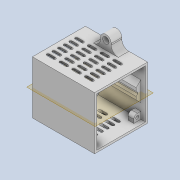
# Autodesk Inventor part: obudowa_WIZ2
Saved by Autodesk Inventor 2021 (Build 250183000, 183)
## iProperties
Created: 2025-11-29
Part Number: obudowa_WIZ2
Material: Generic
Document SubType Name: Modeling
Designer: huber
Density: 1 g/cm^3
Appearance: Default
Author: huber
Autodesk Inventor part; units mm, degrees
ref_plane "YZ Plane" through (0, 0, 0) normal (1, 0, 0) x (0, 1, 0)
ref_plane "XY Plane" through (0, 0, 0) normal (0, 0, 1) x (1, 0, 0)
sketch "Sketch1" plane through (0, 0, 0) normal (1, 0, 0) x (0, 1, 0)
  line L0 (37.5, 37.5) -> (-37.5, 37.5)
  line L1 (-37.5, 37.5) -> (-37.5, -37.5)
  line L2 (-37.5, -37.5) -> (37.5, -37.5)
  line L3 (37.5, -37.5) -> (37.5, 37.5)
  line L4 (37.5, 37.5) -> (-37.5, -37.5) construction
  line L5 (-37.5, 37.5) -> (37.5, -37.5) construction
  line L6 (34.5, 34.5) -> (-34.5, 34.5)
  line L7 (-34.5, 34.5) -> (-34.5, -34.5)
  line L8 (-34.5, -34.5) -> (34.5, -34.5)
  line L9 (34.5, -34.5) -> (34.5, 34.5)
  line L10 (34.5, 34.5) -> (-32.538, -32.538) construction
  line L11 (-34.5, 34.5) -> (32.4964, -32.4964) construction
  line L12 (-52.5, 0) -> (52.5, 0) projected
  line L13 (0, -52.5) -> (0, 52.5) projected
  line L14 (-14, 34.5) -> (-7.5, 28)
  line L15 (-7.5, 28) -> (7.5, 28)
  line L16 (7.5, 28) -> (14, 34.5)
  line L17 (-14, -34.5) -> (-7.5, -28)
  line L18 (-7.5, -28) -> (7.5, -28)
  line L19 (7.5, -28) -> (14, -34.5)
  line L20 (-3.15, 28) -> (-0.9, 30.25)
  line L21 (-0.9, 30.25) -> (0.9, 30.25)
  line L22 (0.9, 30.25) -> (3.15, 28)
  line L23 (-3.15, -28) -> (-0.9, -30.25)
  line L24 (-0.9, -30.25) -> (0.9, -30.25)
  line L25 (0.9, -30.25) -> (3.15, -28)
  point P0 (0, 0)
  dimension "d0" = 75
  dimension "d1" = 75
  dimension "d2" = 3
  dimension "d4" = 45
  dimension "d5" = 60.5
  dimension "d6" = 1.8
  dimension "d7" = 1.8
  dimension "d8" = 56
  dimension "d9" = 15
  dimension "d10" = 15
  dimension "d48" = 3
  dimension "d49" = 3
  dimension "d50" = 3
  constraints: 48 end point, 10 point on line, 6 parallel, 6 perpendicular, 4 horizontal, 2 midpoint, 6 other
  measures "d0" distance of L1.end L2.end
  measures "d1" distance of L0.end L1.end
  measures "d2" distance between parallel lines of L2 L8
  measures "d4" angle of L15 L22
  measures "d5" distance between parallel lines of L21 L24
  measures "d6" distance of L24.end L23.end
  measures "d7" distance of L21.end L20.end
  measures "d8" distance between parallel lines of L18 L15
  measures "d9" distance of L14.end L15.end
  measures "d10" distance of L18.end L17.end
  measures "d48" distance between parallel lines of L9 L3
  measures "d49" distance between parallel lines of L0 L6
  measures "d50" distance between parallel lines of L1 L7
extrude "Extrusion1" add sketch "Sketch1" along normal blind 85 contours L3 L12 L9 L6 L13 L0 | L13 L6 L7 L12 L1 L0 | L3 L2 L13 L8 L9 L12 | L13 L21 L20 L15 L14 L6 | L6 L16 L15 L22 L21 L13 | L12 L7 L8 L13 L2 L1 | L13 L24 L25 L18 L19 L8 | L8 L17 L18 L23 L24 L13
extrude "Extrusion2" add sketch "Sketch1" against normal blind 3
sketch "Sketch3" plane through (85, -37.5, -37.5) normal (0, -1, 0) x (1, 0, 0)
  line L0 (-88, 75) -> (0, 75) projected
  line L1 (-42.5, 75) -> (-42.5, 0) construction
  line L2 (0, 0) -> (-88, 0) projected
  line L3 (0, 75) -> (0, 0) projected
  point P0 (-85, 37.5)
  dimension "d16" = 42.5
  constraints: 2 end point, 2 point on line, 1 vertical
  measures "d16" distance between parallel lines of L3 L1
ref_plane "Work Plane1" through (42.5, -37.5, 37.5) normal (0.7071068, -0.7071068, 0) x (0, 0, -1)
sketch "Sketch5" plane through (42.5, -37.5, 37.5) normal (0.7071068, -0.7071068, 0) x (0, 0, -1)
  line L0 (0, 0) -> (75, 0) construction
  line L1 (37.5, 0) -> (37.5, 3.2791) construction
  line L2 (37.5, 0) -> (37.5, 13.5441)
  line L3 (37.5, 0) -> (37.5, 5) construction
  line L4 (39.5, 0) -> (39.5, 5)
  line L5 (35.5, 5) -> (35.5, 0)
  arc A0 (35.5, 0) -> (39.5, 0) centre (37.5, 0) ccw
  arc A1 (39.5, 5) -> (35.5, 5) centre (37.5, 5) ccw
  point P0 (37.5, -3.5355)
  point P1 (37.5, 2.5)
  dimension "d19" = 4
  dimension "d20" = 5
  constraints: 12 end point, 4 point on circle, 4 tangent, 2 centre point, 2 midpoint, 2 vertical, 1 parallel, 1 point on line
  measures "d19" distance between parallel lines of L4 L5
  measures "d20" distance of L1.start L3.end
extrude "Extrusion3" cut sketch "Sketch5" against normal mid plane 33
pattern_linear "Rectangular Pattern1" count 6 spacing 8 along (0, 0, 1) count 4 spacing 18 along (-1, 0, 0) of "Extrusion3" first direction both ways yes second direction both ways yes
mirror "Mirror1" about plane through (0, 0, 0) normal (0, 1, 0) of "Extrusion3", "Rectangular Pattern1"
sketch "Sketch6" plane through (-3, 0, 0) normal (-1, 0, 0) x (0, 0, 1)
  line L0 (0, 52.5) -> (0, -52.5) projected
  line L1 (-34.5, -14) -> (-34.5, -34.5) projected
  line L2 (-28, -7.5) -> (-34.5, -14) projected
  line L3 (-28, -3.15) -> (-28, -7.5) projected
  line L4 (-30.25, -0.9) -> (-28, -3.15) projected
  line L5 (-30.25, 0.9) -> (-30.25, -0.9) projected
  line L6 (-28, 3.15) -> (-30.25, 0.9) projected
  line L7 (-28, 7.5) -> (-28, 3.15) projected
  line L8 (-34.5, 14) -> (-28, 7.5) projected
  line L9 (-34.5, 34.5) -> (-34.5, 14) projected
  line L10 (34.5, 34.5) -> (-34.5, 34.5) projected
  line L11 (34.5, 14) -> (34.5, 34.5) projected
  line L12 (28, 7.5) -> (34.5, 14) projected
  line L13 (28, 3.15) -> (28, 7.5) projected
  line L14 (30.25, 0.9) -> (28, 3.15) projected
  line L15 (30.25, -0.9) -> (30.25, 0.9) projected
  line L16 (28, -3.15) -> (30.25, -0.9) projected
  line L17 (28, -7.5) -> (28, -3.15) projected
  line L18 (34.5, -14) -> (28, -7.5) projected
  line L19 (34.5, -34.5) -> (34.5, -14) projected
  line L20 (-34.5, -34.5) -> (34.5, -34.5) projected
  point P0 (0, 0)
extrude "Extrusion4" cut sketch "Sketch6" against normal blind 33
ref_plane "Work Plane2" through (78.5, 0, 0) normal (1, 0, 0) x (0, 0, -1)
sketch "Sketch7" plane through (78.5, 0, 0) normal (1, 0, 0) x (0, 0, -1)
  line L0 (37.5, -37.5) -> (37.5, 37.5) projected
  line L1 (37.5, 37.5) -> (-37.5, 37.5) projected
  line L2 (-37.5, 37.5) -> (-37.5, -37.5) projected
  line L3 (-37.5, -37.5) -> (37.5, -37.5) projected
  line L4 (34.5, -34.5) -> (-34.5, -34.5) projected
  line L5 (-34.5, -34.5) -> (-34.5, -14) projected
  line L6 (-34.5, -14) -> (-28, -7.5) projected
  line L7 (-28, -7.5) -> (-28, -3.15) projected
  line L8 (-28, -3.15) -> (-30.25, -0.9) projected
  line L9 (-30.25, -0.9) -> (-30.25, 0.9) projected
  line L10 (-30.25, 0.9) -> (-28, 3.15) projected
  line L11 (-28, 3.15) -> (-28, 7.5) projected
  line L12 (-28, 7.5) -> (-34.5, 14) projected
  line L13 (-34.5, 14) -> (-34.5, 34.5) projected
  line L14 (-34.5, 34.5) -> (34.5, 34.5) projected
  line L15 (34.5, 34.5) -> (34.5, 14) projected
  line L16 (34.5, 14) -> (28, 7.5) projected
  line L17 (28, 7.5) -> (28, 3.15) projected
  line L18 (28, 3.15) -> (30.25, 0.9) projected
  line L19 (30.25, 0.9) -> (30.25, -0.9) projected
  line L20 (30.25, -0.9) -> (28, -3.15) projected
  line L21 (28, -3.15) -> (28, -7.5) projected
  line L22 (28, -7.5) -> (34.5, -14) projected
  line L23 (34.5, -14) -> (34.5, -34.5) projected
  circle A0 centre (-29.5, 29.5) radius 2.15
  line L24 (-25.3431, 29.5) -> (-27.4215, 25.9)
  line L25 (-27.4215, 25.9) -> (-31.5785, 25.9)
  line L26 (-31.5785, 25.9) -> (-33.6569, 29.5)
  line L27 (-33.6569, 29.5) -> (-31.5785, 33.1)
  line L28 (-31.5785, 33.1) -> (-27.4215, 33.1)
  line L29 (-27.4215, 33.1) -> (-25.3431, 29.5)
  line L30 (-34.5, 34.5) -> (34.5, 34.5) projected
  circle A1 centre (-29.5, 29.5) radius 5
  line L31 (-24.5, 29.5) -> (-24.5, 34.5)
  line L32 (-29.5, 24.5) -> (-34.5, 24.5)
  line L33 (-34.5, 14) -> (-34.5, 34.5) projected
  circle A2 centre (29.5, -29.5) radius 5
  line L34 (25.3431, -29.5) -> (27.4215, -25.9)
  line L35 (27.4215, -25.9) -> (31.5785, -25.9)
  line L36 (31.5785, -25.9) -> (33.6569, -29.5)
  line L37 (33.6569, -29.5) -> (31.5785, -33.1)
  line L38 (31.5785, -33.1) -> (27.4215, -33.1)
  line L39 (27.4215, -33.1) -> (25.3431, -29.5)
  circle A3 centre (29.5, -29.5) radius 2.15
  line L40 (29.5, -24.5) -> (34.5, -24.5)
  line L41 (24.5, -29.5) -> (24.5, -34.5)
  line L42 (34.5, -14) -> (34.5, -34.5) projected
  point P0 (0, 0)
  point P1 (-34.5, 24.5)
  point P2 (-34.5, 29.5)
  point P3 (-29.5, 34.5)
  dimension "d33" = 4.3
  dimension "d34" = 5
  dimension "d35" = 5
  dimension "d36" = 7.2
  dimension "d41" = 5
  dimension "d42" = 5
  dimension "d43" = 7.2
  dimension "d44" = 4.3
  constraints: 32 end point, 6 tangent, 4 centre point, 4 coincident, 4 point on circle, 4 point on line, 2 parallel, 2 perpendicular, 1 horizontal, 1 vertical, 26 other
  measures "d33" diameter of A0
  measures "d34" distance from line of L14 A0.centre
  measures "d35" distance from line of L13 A0.centre
  measures "d36" distance between parallel lines of L25 L28
  measures "d41" distance from line of L23 A2.centre
  measures "d42" distance from line of A2.centre L4
  measures "d43" distance between parallel lines of L38 L35
  measures "d44" diameter of A3
extrude "Extrusion5" add sketch "Sketch7" against normal blind 8 contours L41 A2 L4 | A2 L23 L4 | A2 | A2 L40 L23 | L13 A1 L32 | L13 L14 A1 | A1 | L14 L31 A1
extrude "Extrusion6" add sketch "Sketch7" against normal blind 4 contours L24 L25 L26 L27 L28 L29 | L34 L35 L36 L37 L38 L39
ref_plane "Work Plane3" through (0, 37.5, -37.5) normal (0, -0.7071068, -0.7071068) x (1, 0, 0)
sketch "Sketch8" plane through (85, 0, 0) normal (1, 0, 0) x (0, 0, -1)
  line L0 (37.5, -37.5) -> (37.5, 37.5) projected
  line L1 (37.5, -37.5) -> (37.5, 37.5) projected
  line L2 (37.5, 37.5) -> (-37.5, 37.5) projected
  line L3 (-37.5, 37.5) -> (-37.5, -37.5) projected
  line L4 (-37.5, -37.5) -> (37.5, -37.5) projected
  line L5 (34.5, -34.5) -> (-34.5, -34.5) projected
  line L6 (-34.5, -34.5) -> (-34.5, -14) projected
  line L7 (-34.5, -14) -> (-28, -7.5) projected
  line L8 (-28, -7.5) -> (-28, -3.15) projected
  line L9 (-28, -3.15) -> (-30.25, -0.9) projected
  line L10 (-30.25, -0.9) -> (-30.25, 0.9) projected
  line L11 (-30.25, 0.9) -> (-28, 3.15) projected
  line L12 (-28, 3.15) -> (-28, 7.5) projected
  line L13 (-28, 7.5) -> (-34.5, 14) projected
  line L14 (-34.5, 14) -> (-34.5, 34.5) projected
  line L15 (-34.5, 34.5) -> (34.5, 34.5) projected
  line L16 (34.5, 34.5) -> (34.5, 14) projected
  line L17 (34.5, 14) -> (28, 7.5) projected
  line L18 (28, 7.5) -> (28, 3.15) projected
  line L19 (28, 3.15) -> (30.25, 0.9) projected
  line L20 (30.25, 0.9) -> (30.25, -0.9) projected
  line L21 (30.25, -0.9) -> (28, -3.15) projected
  line L22 (28, -3.15) -> (28, -7.5) projected
  line L23 (28, -7.5) -> (34.5, -14) projected
  line L24 (34.5, -14) -> (34.5, -34.5) projected
  line L25 (28, -7.5) -> (34.5, -14) projected
  line L26 (34.5, -14) -> (34.5, 14)
  line L27 (-34.5, -14) -> (-34.5, 14)
  point P0 (0, 0)
  constraints: 4 end point, 1 vertical
extrude "Extrusion8" cut sketch "Sketch8" against normal up to surface (6.5 mm away) contours L23 L22 L21 L20 L19 L18 L17 L26 | L27 L13 L12 L11 L10 L9 L8 L7
sketch "Sketch12" plane through (85, -37.5, -37.5) normal (0, 0, -1) x (-1, 0, 0)
  line L0 (88, 75) -> (0, 75) projected
  line L1 (0, 0) -> (0, 75) projected
  line L2 (0, 0) -> (88, 0) projected
  line L3 (88, 75) -> (88, 0) projected
  line L4 (88, 75) -> (0, 75) projected
  line L5 (44, 75) -> (44, 0)
  circle A0 centre (44, 87) radius 7.5
  line L6 (51.5, 87) -> (51.5, 75)
  line L7 (88, 75) -> (0, 75) projected
  line L8 (36.5, 87) -> (36.5, 75)
  point P0 (85, 37.5)
  dimension "d80" = 15
  dimension "d81" = 12
  constraints: 6 end point, 3 point on line, 2 midpoint, 2 perpendicular, 2 point on circle, 2 tangent, 1 centre point, 1 parallel
  measures "d80" diameter of A0
  measures "d81" distance from line of A0.centre L0
extrude "Extrusion10" add sketch "Sketch12" against normal blind 15 contours L0 L8 A0 L6 | A0
fillet "Fillet3" radius 10 2 edges at (33.5, 37.5, -30) (48.5, 37.5, -30)
sketch "Sketch13" plane through (85, -37.5, -22.5) normal (0, 0, 1) x (1, 0, 0)
  line L0 (-36.5, 85) -> (-36.5, 87) projected
  arc A0 (-36.5, 87) -> (-51.5, 87) centre (-44, 87) ccw projected
  line L1 (-51.5, 87) -> (-51.5, 85) projected
  arc A1 (-61.5, 75) -> (-51.5, 85) centre (-61.5, 85) ccw projected
  line L2 (-26.5, 75) -> (-61.5, 75) projected
  arc A2 (-36.5, 85) -> (-26.5, 75) centre (-26.5, 85) ccw projected
  point P0 (-85, 37.5)
  constraints: 1 coincident
hole "Hole2" at (41, 49.5, -22.5) direction (0, 0, -1) diameter 9 end through all clearance for "Socket Head Cap Screw ISO 4762" size "M8" standard "ISO"
mirror "Mirror6" about plane through (0, 0, 0) normal (0, 1, 0) of "Fillet3", "Extrusion10", "Hole2"
equation "\"d7\" = d6"
equation "\"d10\" = d9"
equation "\"d43\" = d36"
body "Solid1"
